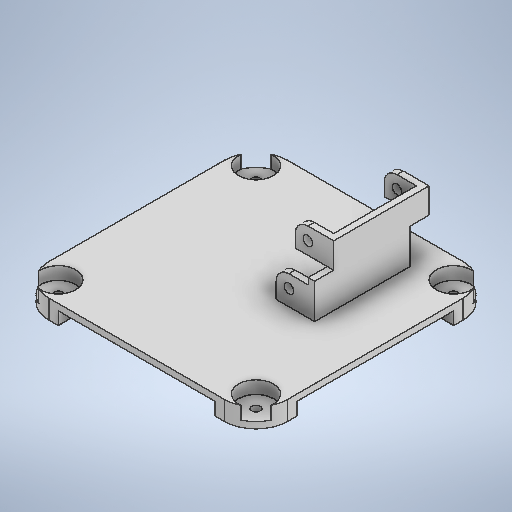
# Autodesk Inventor part: housing_shaft_link_base_2
Saved by Autodesk Inventor 2025 (Build 290162000, 162)
## iProperties
Created: 2025-10-03
Part Number: housing_shaft_link_base_2
Material: 一般
Document SubType Name: Modeling
Designer: sooo1
Density: 1 g/cm^3
Appearance: 既定
Author: sooo1
Autodesk Inventor part; units mm, degrees
ref_plane "YZ Plane" through (0, 0, 0) normal (1, 0, 0) x (0, 1, 0)
ref_plane "XZ Plane" through (0, 0, 0) normal (0, 1, 0) x (-1, 0, 0)
ref_plane "XY Plane" through (0, 0, 0) normal (0, 0, 1) x (1, 0, 0)
sketch "スケッチ2" plane through (0, 0, 0) normal (0, 0, 1) x (1, 0, 0)
  line L0 (-4, 4) -> (8.1, 4)
  line L1 (8.1, 4) -> (8.1, -4)
  line L2 (8.1, -4) -> (-4, -4)
  line L3 (-4, -4) -> (-4, 4)
  line L4 (2.05, 4) -> (2.05, -4) construction
  line L5 (-4, 0) -> (8.1, 0) construction
  circle A0 centre (0, 0) radius 1.5
  line L6 (0, 0) -> (0, -10) construction
  circle A1 centre (0, -10) radius 1.5
  line L7 (6.1, 4) -> (6.1, -4)
  line L8 (-4, -4) -> (-4, -15)
  line L9 (-4, -15) -> (8.1, -15)
  line L10 (8.1, -15) -> (8.1, -4)
  line L11 (6.1, -4) -> (6.1, -15)
  line L12 (-4, -6) -> (6.1, -6)
  line L13 (-4, 4) -> (-6, 4)
  line L14 (-6, 4) -> (-6, -15)
  line L15 (-6, -15) -> (-4, -15)
  line L16 (-4, -4) -> (-6, -4)
  line L17 (-4, -6) -> (-6, -6)
  line L18 (6.1, -6) -> (8.1, -6)
  line L19 (8.1, -15) -> (37.1447, -15)
  line L20 (-6, -15) -> (-30.9963, -15)
  circle A2 centre (27.1, 4) radius 19
  circle A3 centre (-25, 4) radius 19
  circle A4 centre (17.1, -6) radius 9
  circle A5 centre (-15, -6) radius 9
  point P0 (-25, -15)
  point P1 (-15, -15)
  point P2 (17.1, -15)
  dimension "d1" = 3
  dimension "d2" = 3
  dimension "d3" = 10
  dimension "d4" = 4
  dimension "d5" = 8.1
  dimension "d6" = 8
  dimension "d7" = 2
  dimension "d8" = 5
  dimension "d21" = 4
  dimension "d84" = 2
  dimension "d91" = 38
  dimension "d92" = 18
  constraints: 42 end point, 10 point on line, 9 perpendicular, 8 tangent, 6 centre point, 5 horizontal, 4 midpoint, 2 coincident, 2 equal radius, 2 parallel, 2 vertical
  measures "d1" diameter of A0
  measures "d2" diameter of A1
  measures "d3" distance of L6.start L6.end
  measures "d4" distance from line of L3 point (0, 0)
  measures "d5" distance from line of L1 point (0, 0)
  measures "d6" distance of L0.end L1.end
  measures "d7" distance between parallel lines of L1 L7
  measures "d8" distance from line of L9 A1.centre
  measures "d21" distance from line of L6.end L12
  measures "d84" distance of L0.start L13.end
  measures "d91" diameter of A2
  measures "d92" diameter of A4
extrude "押し出し1" add sketch "スケッチ2" along normal mid plane 30 contours L0 L7 L2 L3 | L0 L1 L2 L7
extrude "押し出し2" cut sketch "スケッチ2" along normal mid plane 26 contours L0 L7 L2 L3
ref_plane "作業平面1" through (0, 0, 14) normal (0, 0, 1) x (1, 0, 0)
extrude "押し出し3" add sketch "スケッチ2" along normal blind 6 and the other way blind 24 from surface at 15 contours L2 L11 L12 L8 | L2 L10 L18 L11 | L12 L11 L9 L8 | L18 L10 L9 L11
extrude "押し出し4" cut sketch "スケッチ2" along normal blind 4 and the other way blind 22 from surface at 15 contours L2 L11 L12 L8 | L12 L11 L9 L8
extrude "押し出し5" cut sketch "スケッチ2" along normal through all both and the other way through all contours L2 L11 L12 L8
sketch "スケッチ3" plane through (-4, -15, -9) normal (0, -1, 0) x (1, 0, 0)
  line L0 (-28, -6) -> (15, -6)
  line L1 (15, -6) -> (15, 41)
  line L2 (15, 41) -> (-28, 41)
  line L3 (-28, 41) -> (-28, -6)
  line L4 (-28, -6) -> (15, 41) construction
  line L5 (15, -6) -> (-28, 41) construction
  line L6 (12.1, 0) -> (12.1, 30) construction
  line L7 (0, 24) -> (10.1, 24) construction
  line L8 (-43.5, 51.2) -> (-43.5, 62.5)
  line L9 (-43.5, 62.5) -> (26.5, 62.5)
  line L10 (26.5, 62.5) -> (26.5, 51.2)
  line L11 (-28, 41) -> (-28, 51.2)
  line L12 (-28, 51.2) -> (-43.5, 51.2)
  line L13 (15, 41) -> (15, 51.2)
  line L14 (15, 51.2) -> (26.5, 51.2)
  line L15 (-28, -6) -> (-28, 5.2)
  line L16 (-28, 5.2) -> (-43.5, 5.2)
  line L17 (-43.5, 5.2) -> (-43.5, -7.5)
  line L18 (-43.5, -7.5) -> (26.5, -7.5)
  line L19 (26.5, -7.5) -> (26.5, 5.2)
  line L20 (26.5, 5.2) -> (15, 5.2)
  line L21 (-43.5, 56.85) -> (26.5, 56.85) construction
  line L22 (-43.5, -1.15) -> (26.5, -1.15) construction
  circle A0 centre (-37.65, -1.15) radius 1.5
  line L23 (-8.5, -7.5) -> (-8.5, 62.5) construction
  circle A1 centre (20.65, -1.15) radius 1.5
  circle A2 centre (-37.65, 56.85) radius 1.5
  line L24 (-37.65, -1.15) -> (-37.65, 56.85) construction
  circle A3 centre (20.65, 56.85) radius 1.5
  line L25 (15, -6) -> (15, -7.5)
  line L26 (-28, -6) -> (-28, -7.5)
  line L27 (-28, 51.2) -> (15, 51.2)
  line L28 (-28, 51.2) -> (-28, 62.5)
  line L29 (15, 51.2) -> (15, 62.5)
  line L30 (-37.65, 27.85) -> (33.8056, 27.85) construction
  line L31 (-23.5, -7.5) -> (6.5, -7.5) construction
  line L32 (6.5, -7.5) -> (6.5, 2.5)
  line L33 (6.5, 2.5) -> (-23.5, 2.5)
  line L34 (-23.5, 2.5) -> (-23.5, -7.5)
  line L35 (-23.5, -7.5) -> (6.5, 2.5) construction
  line L36 (6.5, -7.5) -> (-23.5, 2.5) construction
  line L37 (6.5, 63.2) -> (6.5, 53.2)
  line L38 (6.5, 53.2) -> (-23.5, 53.2)
  line L39 (-23.5, 53.2) -> (-23.5, 63.2)
  circle A4 centre (20.65, -1.15) radius 5
  circle A5 centre (-37.65, -1.15) radius 5
  circle A6 centre (-37.65, 56.85) radius 5
  circle A7 centre (20.65, 56.85) radius 5
  line L40 (-16.1, 35.45) -> (-0.9, 35.45)
  line L41 (-0.9, 35.45) -> (-0.9, 20.25)
  line L42 (-0.9, 20.25) -> (-16.1, 20.25)
  line L43 (-16.1, 20.25) -> (-16.1, 35.45)
  line L44 (-16.1, 35.45) -> (-0.9, 20.25) construction
  line L45 (-0.9, 35.45) -> (-16.1, 20.25) construction
  line L46 (-46.05, -9.7) -> (29.05, -9.7)
  line L47 (29.05, -9.7) -> (29.05, 65.4)
  line L48 (29.05, 65.4) -> (-46.05, 65.4)
  line L49 (-46.05, 65.4) -> (-46.05, -9.7)
  line L50 (-46.05, -9.7) -> (29.05, 65.4) construction
  line L51 (29.05, -9.7) -> (-46.05, 65.4) construction
  circle A8 centre (-8.5, 27.85) radius 44 construction
  circle A9 centre (-39.6127, 58.9627) radius 1.35
  circle A10 centre (-39.6127, -3.2627) radius 1.35
  circle A11 centre (22.6127, -3.2627) radius 1.35
  circle A12 centre (22.6127, 58.9627) radius 1.35
  point P0 (4, 9)
  point P1 (-6.5, 17.5)
  point P2 (-28, 5.2)
  point P3 (-8.5, -2.5)
  point P4 (6.5, 62.5)
  point P5 (-23.5, 62.5)
  point P6 (-23.5, -7.5)
  point P7 (-8.5, 27.85)
  dimension "d66" = 88
  dimension "d25" = 2.9
  dimension "d26" = 17
  dimension "d27" = 43
  dimension "d28" = 47
  dimension "d32" = 70
  dimension "d33" = 11.5
  dimension "d34" = 70
  dimension "d35" = 58
  dimension "d36" = 1.5
  dimension "d37" = 3
  dimension "d38" = 58.3
  dimension "d44" = 6.35
  dimension "d51" = 10
  dimension "d52" = 30
  dimension "d58" = 10
  dimension "d61" = 15.2
  dimension "d64" = 75.1
  dimension "d65" = 75.1
  dimension "d67" = 2.7
  dimension "d70" = 360
  constraints: 100 end point, 18 perpendicular, 15 midpoint, 14 point on line, 12 centre point, 8 parallel, 6 horizontal, 6 symmetric about line, 5 coincident, 5 vertical, 4 equal radius, 2 equal length, 1 collinear, 14 other
  measures "d25" distance between parallel lines of L1 L6
  measures "d26" distance between parallel lines of L2 L7
  measures "d27" distance of L1.end L2.end
  measures "d28" distance of L0.end L1.end
  measures "d32" distance of L17.end L18.end
  measures "d33" distance of L19.end L20.end
  measures "d34" distance between parallel lines of L9 L18
  measures "d35" distance between parallel lines of L21 L22
  measures "d36" distance between parallel lines of L0 L18
  measures "d37" diameter of A0
  measures "d38" diameter of L24.start L23
  measures "d44" distance between parallel lines of L18 L22
  measures "d51" distance of L31.end L32.end
  measures "d52" distance of L31.start L31.end
  measures "d58" diameter of A4
  measures "d61" distance of L40.start L40.end
  measures "d64" distance of L48.end L46.start
  measures "d65" distance of L46.start L46.end
  measures "d67" diameter of A9
extrude "押し出し6" add sketch "スケッチ3" along normal blind 2 contours L3 L2 L1 L0 L32 L33 L34 | L34 L33 L32 L0 | L40 L41 L42 L43
extrude "押し出し7" add sketch "スケッチ3" along normal blind 2 contours L26 L18 L17 L16 L3 | L0 L34 L18 L26 | L0 L32 L18 L34 | L0 L25 L18 L32 | L11 L27 L13 L2 | L1 L20 L19 L18 L25 | L28 L9 L39 L38 L37 L29 L27 | L12 L8 L9 L28 | L29 L9 L10 L14 | L9 L37 L38 L39 | A4 | A5 | A6 | A7 | A9 | A10 | A11 | A12
extrude "押し出し13" add sketch "スケッチ3" along normal blind 2 contours A0 | A1 | A2 | A3 | L49 L48 L47 L46
extrude "押し出し14" cut sketch "スケッチ3" along normal blind 2 contours A9 | A10 | A11 | A12
ref_plane "作業平面3" through (6.1, -4, 1) normal (0, 0, 1) x (1, 0, 0)
ref_plane "作業平面4" through (0, 0, -5) normal (0, 0, 1) x (1, 0, 0)
fillet "フィレット6" radius 10 4 edges at (25.05, -16, -18.7) (-50.05, -16, -18.7) (25.05, -16, 56.4) (-50.05, -16, 56.4)
sketch "スケッチ4" plane through (-4, -15, -9) normal (0, 1, 0) x (1, 0, 0)
  line L0 (12.1, -10) -> (-11, -10) projected
  line L1 (8, -1.5) -> (-18, -1.5)
  line L2 (8, 4.5) -> (-18, 4.5)
  line L3 (2.5, -12) -> (5.5, -12) projected
  line L4 (2.5, -10) -> (5.5, -10) projected
  line L5 (4, -12) -> (4, 4.5) construction
  circle A0 centre (4, 1.5) radius 2
  line L6 (8, -1.5) -> (8, 4.5)
  line L7 (0, -1.5) -> (0, 4.5)
  line L8 (-10, -1.5) -> (-10, 4.5)
  circle A1 centre (-14, 1.5) radius 2
  line L9 (-18, -1.5) -> (-18, 4.5)
  arc A2 (19.05, -65.4) -> (29.05, -55.4) centre (19.05, -55.4) ccw projected
  arc A3 (-46.05, -55.4) -> (-36.05, -65.4) centre (-36.05, -55.4) ccw projected
  arc A4 (29.05, -0.3) -> (19.05, 9.7) centre (19.05, -0.3) ccw projected
  arc A5 (-36.05, 9.7) -> (-46.05, -0.3) centre (-36.05, -0.3) ccw projected
  circle A6 centre (19.05, -55.4) radius 10
  circle A7 centre (19.05, -0.3) radius 10
  circle A8 centre (-36.05, -0.3) radius 10
  circle A9 centre (-36.05, -55.4) radius 10
  line L10 (29.05, -3.2) -> (-46.05, -3.2)
  line L11 (-46.05, -55.4) -> (-46.05, -0.3) projected
  line L12 (-36.05, 9.7) -> (19.05, 9.7) projected
  line L13 (16.15, 9.7) -> (16.15, -65.4)
  line L14 (19.05, -65.4) -> (-36.05, -65.4) projected
  line L15 (19.05, -55.4) -> (-36.05, -0.3) construction
  line L16 (-33.15, -65.4) -> (-33.15, 9.7)
  line L17 (-46.7591, -52.5) -> (29.05, -52.5)
  line L18 (29.05, -0.3) -> (29.05, -55.4) projected
  circle A10 centre (22.6127, -58.9627) radius 1.35 projected
  circle A11 centre (-39.6127, -58.9627) radius 1.35 projected
  circle A12 centre (-39.6127, 3.2627) radius 1.35 projected
  circle A13 centre (22.6127, 3.2627) radius 1.35 projected
  circle A14 centre (-39.6127, 3.2627) radius 5.5
  circle A15 centre (-39.6127, -58.9627) radius 5.5
  circle A16 centre (22.6127, -58.9627) radius 5.5
  circle A17 centre (22.6127, 3.2627) radius 5.5
  line L19 (15.15, -10) -> (13.15, -10) construction
  line L20 (13.15, -10) -> (13.15, 9.7)
  line L21 (13.15, 9.7) -> (15.15, 9.7) construction
  line L22 (15.15, 9.7) -> (15.15, -10)
  line L23 (15.15, -10) -> (13.15, 9.7) construction
  line L24 (13.15, -10) -> (15.15, 9.7) construction
  line L25 (-18.5, -1.5) -> (-20.5, -1.5)
  line L26 (-20.5, -1.5) -> (-20.5, 9.7)
  line L27 (-20.5, 9.7) -> (-18.5, 9.7) construction
  line L28 (-18.5, 9.7) -> (-18.5, -1.5)
  line L29 (-18.5, -1.5) -> (-20.5, 9.7) construction
  line L30 (-20.5, -1.5) -> (-18.5, 9.7) construction
  line L31 (8, 4.5) -> (21.15, 4.5)
  line L32 (21.15, 4.5) -> (21.15, -1.5)
  line L33 (21.15, -1.5) -> (8, -1.5)
  line L34 (-18, 4.5) -> (-26.5, 4.5)
  line L35 (-26.5, 4.5) -> (-26.5, -1.5)
  line L36 (-26.5, -1.5) -> (-18, -1.5)
  line L37 (-20.5, -1.5) -> (-26.5, 4.5) construction
  line L38 (-26.5, -1.5) -> (-20.5, 4.5) construction
  circle A18 centre (-23.5, 1.5) radius 1.25
  line L39 (21.15, -1.5) -> (15.15, 4.5) construction
  line L40 (21.15, 4.5) -> (15.15, -1.5) construction
  circle A19 centre (18.15, 1.5) radius 1.25
  line L41 (15.15, -10) -> (12.1, -10)
  line L42 (15.15, -10) -> (15.15, -12)
  line L43 (15.15, -12) -> (12.1, -12)
  line L44 (12.1, 0) -> (12.1, -30) projected
  point P0 (4, -9)
  point P1 (-8.5, -27.85)
  point P2 (-33.15, -3.2)
  point P3 (16.15, -3.2)
  point P4 (16.15, -52.5)
  point P5 (-33.15, -52.5)
  point P6 (-46.05, -52.5)
  point P7 (14.15, -0.15)
  point P8 (-19.5, 4.1)
  point P9 (-18.5, 9.7)
  point P10 (-20.5, -1.5)
  point P11 (-20.5, 4.5)
  point P12 (15.15, -1.5)
  point P13 (13.15, -1.5)
  point P14 (13.15, 4.5)
  point P15 (-18.5, 4.5)
  point P16 (12.1, -28)
  dimension "d99" = 8.5
  dimension "d100" = 6
  dimension "d101" = 4
  dimension "d102" = 3
  dimension "d103" = 8
  dimension "d104" = 4
  dimension "d107" = 18
  dimension "d117" = 2.9
  dimension "d118" = 2.9
  dimension "d119" = 2.9
  dimension "d120" = 2.9
  dimension "d125" = 360
  dimension "d130" = 11
  dimension "d131" = 2
  dimension "d132" = 5.15
  dimension "d133" = 2
  dimension "d134" = 0.5
  dimension "d137" = 6
  dimension "d138" = 6
  dimension "d139" = 2.5
  dimension "d140" = 2.5
  dimension "d143" = 2
  constraints: 74 end point, 19 point on line, 15 perpendicular, 12 centre point, 9 coincident, 8 midpoint, 7 parallel, 6 collinear, 4 concentric, 4 horizontal, 1 vertical, 17 other
  measures "d99" distance between parallel lines of L0 L1
  measures "d100" distance between parallel lines of L2 L1
  measures "d101" diameter of A0
  measures "d102" distance from line of L2 A0.centre
  measures "d103" distance between parallel lines of L6 L7
  measures "d104" distance between parallel lines of L6 L5
  measures "d107" distance of L6.start L8.start
  measures "d117" distance from line of L10 A7.centre
  measures "d118" distance from line of A4.centre L13
  measures "d119" distance from line of L17 A3.centre
  measures "d120" distance from line of L16 A9.centre
  measures "d130" diameter of A14
  measures "d131" distance of L20.end L21.end
  measures "d132" distance between parallel lines of L6 L20
  measures "d133" distance of L25.start L25.end
  measures "d134" distance between parallel lines of L28 L9
  measures "d137" distance between parallel lines of L35 L26
  measures "d138" distance between parallel lines of L22 L32
  measures "d139" diameter of A18
  measures "d140" diameter of A19
  measures "d143" distance between parallel lines of L19 L43
extrude "押し出し26" add sketch "スケッチ4" against normal blind 4 from surface at -2 contours L10 A8 A5 A14 L16 | L13 L12 A7 | A7 A4 A17 L31 L13 | L31 A17 A19 L33 L13 | L10 L11 A8 | A8 L12 L16 | L33 A17 A4 A7 L10 L13 | L31 L32 L33 A17 A19 | A17 A4 L33 L32 L31 | L17 L16 A9 A3 A15 | A9 L11 L17 | A19 A17 | A17 A19 | A7 L18 L10 | A5 A14 | L16 L14 A9 | L17 L18 A6 | A6 A2 A16 L13 L17 | A6 L14 L13 | A15 A3 | A2 A16 picked at (-40.819, 6.9422) picked at (-40.819, -62.6422) picked at (23.819, -62.6422)
extrude "押し出し34" cut sketch "スケッチ4" along normal blind 10 and the other way blind 4 from surface at 0 contours L31 L32 L33 A17 A19 | A17 A4 L33 L32 L31 | A17 A4 | A19 A17 | A14 A5 | A5 A14 | A15 A3 | A3 A15 | A16 A2 | A2 A16 | A10 | A11 | A12 | A13 picked at (18.0906, 1.5264)
fillet "フィレット9" radius 4 4 edges at (-4, -6, 20) (-4, 4, 14) (-4, 4, -14) (-4, -6, -8)
